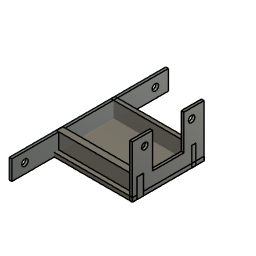
SupportMoteurCV v5 (Autodesk Fusion 360 design; units mm, degrees)
Autodesk Fusion 360 part; units mm, degrees
box "BoitePrimitive1" add length 15 width 120 height 5 placed x (0, -1, 0) y (0, 0, -1) z (1, 0, 0) at (0, 35, 40) makes body 1
move_face "DéplacerFace1" by (-2, 0, -10) 1 faces at (5, 30, -40) on bodies 1
copy_body "Copier/Coller des corps1" bodies 1 makes body 2
move_body "Déplacer1" bodies 2 to x (1, 0, 0) y (0, 1, 0) z (0, 0, 1) at (56, 0, 0)
move_face "DéplacerFace2" by (0, 0, -32.5) 1 faces at (57, 25, 40) on bodies 2
move_face "DéplacerFace3" by (0, 0, 32.5) 1 faces at (57, 25, -80) on bodies 2
move_face "DéplacerFace4" by (0, 15, 0) 1 faces at (57, 35, -29.1667) on bodies 2
box "BoitePrimitive2" add length 55 width 62 height 3 placed x (0, 0, 1) y (1, 0, 0) z (0, 1, 0) at (-4.8215, 0, -6.5989) separate body makes body 3
move_face "DéplacerFace5" by (0, 0, -25) 1 faces at (36.5118, 3, 11.7344) on bodies 3
move_face "DéplacerFace6" by (0, 0, -10) 1 faces at (36.5118, 3, 11.7344) on bodies 3
move_body "Déplacer2" bodies 3 to x (1, 0, 0) y (0, 1, 0) z (0, 0, 1) at (0, 0, -40)
move_body "Déplacer3" bodies 1 to x (1, 0, 0) y (0, 1, 0) z (0, 0, 1) at (-19.4846, -18.5661, 2.6856)
move_face "DéplacerFace7" by (0, -10, 0) 1 faces at (56, 40, -29.1667) on bodies 2
move_body "Déplacer4" bodies 2 to x (1, 0, 0) y (0, 1, 0) z (0, 0, 1) at (0, -10, 0)
move_face "DéplacerFace8" by (0, -15, 0) 1 faces at (56, 30, -29.1667) on bodies 2
move_body "Déplacer5" bodies 2 to x (1, 0, 0) y (0, 1, 0) z (0, 0, 1) at (0, -10, 0)
move_body "Déplacer6" bodies 2 to x (1, 0, 0) y (0, 1, 0) z (0, 0, 1) at (1.5, 0, 0)
move_body "Déplacer7" bodies 2 to x (1, 0, 0) y (0, 1, 0) z (0, 0, 1) at (0, 0, 1)
move_body "Déplacer8" bodies 1 to x (1, 0, 0) y (0, 1, 0) z (0, 0, 1) at (12, 0, 0)
move_body "Déplacer9" bodies 1 to x (1, 0, 0) y (0, 1, 0) z (0, 0, 1) at (0, -2, 0)
move_face "DéplacerFace9" by (-1, 0, 0) 1 faces at (-4.4846, 9.4339, -37.3144) on bodies 1
move_body "Déplacer10" bodies 1 to x (1, 0, 0) y (0, 1, 0) z (0, 0, 1) at (0, 1, 0)
move_face "DéplacerFace10" by (1, 0, 0) 1 faces at (-6.8179, 15.4339, 2.6856) on bodies 1
move_body "Déplacer11" bodies 1 to x (1, 0, 0) y (0, 1, 0) z (0, 0, 1) at (1, 0, 0)
move_body "Déplacer12" bodies 1 to x (1, 0, 0) y (0, 1, 0) z (0, 0, 1) at (0, 0, -5)
move_body "Déplacer13" bodies 1 to x (1, 0, 0) y (0, 1, 0) z (0, 0, 1) at (0, -1, 0)
move_body "Déplacer14" bodies 1 to x (1, 0, 0) y (0, 1, 0) z (0, 0, 1) at (-1, 0, 0)
move_body "Déplacer15" bodies 1 to x (1, 0, 0) y (0, 1, 0) z (0, 0, 1) at (0, 1, 0)
move_body "Déplacer16" bodies 1 to x (1, 0, 0) y (0, 1, 0) z (0, 0, 1) at (0.5, 0, 0)
move_body "Déplacer17" bodies 2 to x (1, 0, 0) y (0, 1, 0) z (0, 0, 1) at (-0.5, 0, 0)
move_body "Déplacer18" bodies 2 to x (1, 0, 0) y (0, 1, 0) z (0, 0, 1) at (0.25, 0, 0)
move_body "Déplacer19" bodies 1 to x (1, 0, 0) y (0, 1, 0) z (0, 0, 1) at (0, 0, 5)
move_body "Déplacer20" bodies 1 to x (1, 0, 0) y (0, 1, 0) z (0, 0, 1) at (0, 0, -0.637)
move_body "Déplacer21" bodies 1 to x (1, 0, 0) y (0, 1, 0) z (0, 0, 1) at (0, -0.25, 0)
move_body "Déplacer22" bodies 1 to x (1, 0, 0) y (0, 1, 0) z (0, 0, 1) at (0, -0.1, 0)
move_body "Déplacer23" bodies 1 to x (1, 0, 0) y (0, 1, 0) z (0, 0, 1) at (0, -0.1, 0)
move_body "Déplacer24" bodies 1 to x (1, 0, 0) y (0, 1, 0) z (0, 0, 1) at (0.1, 0, 0)
move_body "Déplacer25" bodies 1 to x (1, 0, 0) y (0, 1, 0) z (0, 0, 1) at (0.1, 0, 0)
move_body "Déplacer26" bodies 2 to x (1, 0, 0) y (0, 1, 0) z (0, 0, 1) at (-0.05, 0, 0)
move_body "Déplacer27" bodies 2 to x (1, 0, 0) y (0, 1, 0) z (0, 0, 1) at (-0.02, 0, 0)
move_body "Déplacer28" bodies 1 to x (1, 0, 0) y (0, 1, 0) z (0, 0, 1) at (0, 0, -1.147)
move_face "DéplacerFace11" by (-2, 0, 0) 1 faces at (60.18, 20, -28.1667) on bodies 2
move_face "DéplacerFace12" by (1, 0, 0) 1 faces at (58.18, 20, -28.1667) on bodies 2
move_body "Déplacer29" bodies 2 to x (1, 0, 0) y (0, 1, 0) z (0, 0, 1) at (-11.58, 0, 0)
move_body "Déplacer30" bodies 2 to x (1, 0, 0) y (0, 1, 0) z (0, 0, 1) at (7.578, 0, 0)
move_face "DéplacerFace13" by (-1.963, 0, 0) 1 faces at (57.1785, 1, -9.9323) on bodies 3
move_body "Déplacer31" bodies 3 to x (1, 0, 0) y (0, 1, 0) z (0, 0, 1) at (-2, 0, 0)
move_body "Déplacer32" bodies 3 to x (1, 0, 0) y (0, 1, 0) z (0, 0, 1) at (-10, 0, 0)
move_face "DéplacerFace14" by (2, 0, 0) 1 faces at (43.2155, 1, -9.9323) on bodies 3
move_body "Déplacer33" bodies 3 to x (1, 0, 0) y (0, 1, 0) z (0, 0, 1) at (10, 0, 0)
form "Forme1" [no effect]
sketch "Esquisse3" plane through (-6.7846, 0, 0) normal (-1, 0, 0) x (0, 0, 1)
  line L0 (-79.0984, -0.0161) -> (40.9016, -0.0161)
  line L1 (40.9016, -0.0161) -> (40.9016, 14.9839)
  line L2 (40.9016, 14.9839) -> (-79.0984, 14.9839)
  line L3 (-79.0984, 14.9839) -> (-79.0984, -0.0161)
cylinder "CylindrePrimitive1" add diameter 5 height 10 placed x (0, 0, 1) y (0, 1, 0) z (-1, 0, 0) at (-6.7846, 7.5663, -73.4959) bodies 1
delete_face "DeleteFace1" 1 faces at (-13.4512, 7.3174, -71.0084) on bodies 1
hole "Perçage1" at (-6.7846, 7.4839, -69.0984) direction (1, 0, 0) diameter 5 depth 14 tip angle 180 bodies 1
hole "Perçage2" at (-6.7846, 7.4839, 30.9016) direction (1, 0, 0) diameter 5 depth 14 tip angle 180 bodies 1
box "BoitePrimitive3" cut length 15 width 62 height 5 placed x (0, 1, 0) y (-1, 0, 0) z (0, 0, 1) at (55.4727, -0.0139, 0) bodies 1 2 3
box "BoitePrimitive4" add length 15 width 62 height 5 placed x (0, 1, 0) y (-1, 0, 0) z (0, 0, 1) at (55, 0, 0) separate body makes body 4
move_body "Déplacer34" bodies 4 to x (1, 0, 0) y (0, 1, 0) z (0, 0, 1) at (0.4, 0, 0)
move_body "Déplacer35" bodies 4 to x (1, 0, 0) y (0, 1, 0) z (0, 0, 1) at (-0.1, 0, 0)
move_body "Déplacer36" bodies 4 to x (1, 0, 0) y (0, 1, 0) z (0, 0, 1) at (0.1, 0, 0)
move_body "Déplacer37" bodies 4 to x (1, 0, 0) y (0, 1, 0) z (0, 0, 1) at (-0.1, 0, 0)
copy_body "Copier/Coller des corps2" bodies 4 makes body 5
move_body "Déplacer38" bodies 5 to x (1, 0, 0) y (0, 1, 0) z (0, 0, 1) at (0, 0, -42)
box "BoitePrimitive5" cut length 15 width 24 height -10 placed x (0, 1, 0) y (0, 0, 1) z (1, 0, 0) at (55.178, 15, -31) bodies 2
move_face "DéplacerFace15" by (0, -2, 0) 1 faces at (53.8447, 15, -23) on bodies 2
move_face "DéplacerFace16" by (0, 0, 2) 1 faces at (34.6333, 5, -42) on bodies 5
move_face "DéplacerFace17" by (0, 7, 0) 1 faces at (53.8447, 30, 3.3333) on bodies 2
move_face "DéplacerFace18" by (0, 7, 0) 1 faces at (53.8447, 30, -36.1667) on bodies 2
move_face "DéplacerFace19" by (0, -5, 0) 1 faces at (53.8447, 37, 3.3333) on bodies 2
move_face "DéplacerFace20" by (0, -5, 0) 1 faces at (53.8447, 37, -36.1667) on bodies 2
move_face "DéplacerFace21" by (0, 8, 0) 1 faces at (53.8447, 32, -36.1667) on bodies 2
move_face "DéplacerFace22" by (0, 8, 0) 1 faces at (53.8447, 32, 3.3333) on bodies 2
hole "Perçage9" at (55.178, 32.5, -1) direction (-1, 0, 0) diameter 5 depth 25 tip angle 118 bodies 2
hole "Perçage10" at (55.178, 32.5, -37) direction (-1, 0, 0) diameter 5 depth 25 tip angle 118 bodies 2
